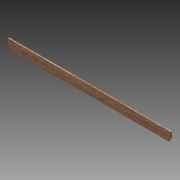
# Autodesk Inventor part: TussenPalet
Saved by Autodesk Inventor 2015 (Build 190159000, 159)
## iProperties
Created: 2016-01-12
Part Number: TussenPalet
Material: Generic
Document SubType Name: Modeling
Designer: david
Density: 1 g/cm^3
Appearance: Birch - Natural Polished
Author: david
Autodesk Inventor part; units mm, degrees
ref_plane "YZ Plane" through (0, 0, 0) normal (1, 0, 0) x (0, 1, 0)
ref_plane "XZ Plane" through (0, 0, 0) normal (0, 1, 0) x (-1, 0, 0)
ref_plane "XY Plane" through (0, 0, 0) normal (0, 0, 1) x (1, 0, 0)
sketch "Sketch1" plane through (0, 0, 0) normal (0, 1, 0) x (-1, 0, 0)
  line L0 (-167.5, 12.5) -> (167.5, 12.5)
  line L1 (167.5, 12.5) -> (167.5, -12.5)
  line L2 (167.5, -12.5) -> (-167.5, -12.5)
  line L3 (-167.5, -12.5) -> (-167.5, 12.5)
  line L4 (-167.5, 12.5) -> (167.5, -12.5) construction
  line L5 (167.5, 12.5) -> (-167.5, -12.5) construction
  line L6 (-171, 6.5) -> (171, 6.5)
  line L7 (171, 6.5) -> (171, -6.5)
  line L8 (171, -6.5) -> (-171, -6.5)
  line L9 (-171, -6.5) -> (-171, 6.5)
  line L10 (-171, 6.5) -> (171, -6.5) construction
  line L11 (171, 6.5) -> (-171, -6.5) construction
  point P0 (0, 0)
  dimension "d0" = 335
  dimension "d1" = 25
  dimension "d2" = 342
  dimension "d3" = 13
  constraints: 24 end point, 4 midpoint, 4 parallel, 2 horizontal, 2 perpendicular
  measures "d0" distance of L1.end L2.end
  measures "d1" distance of L0.end L1.end
  measures "d2" distance of L7.end L8.end
  measures "d3" distance of L6.end L7.end
extrude "Extrusion1" add sketch "Sketch1" along normal blind 3
sketch "Sketch2" plane through (0, 3, 0) normal (0, 1, 0) x (1, 0, 0)
  line L0 (167.5, -6.5) -> (-167.5, -6.5)
  line L1 (-167.5, -6.5) -> (-167.5, -12.5)
  line L2 (-167.5, -12.5) -> (167.5, -12.5)
  line L3 (167.5, -12.5) -> (167.5, -6.5)
  point P0 (0, 0)
  constraints: 8 end point, 2 parallel, 1 horizontal, 1 perpendicular
extrude "Extrusion2" cut sketch "Sketch2" against normal blind 3
body "Solid1"
